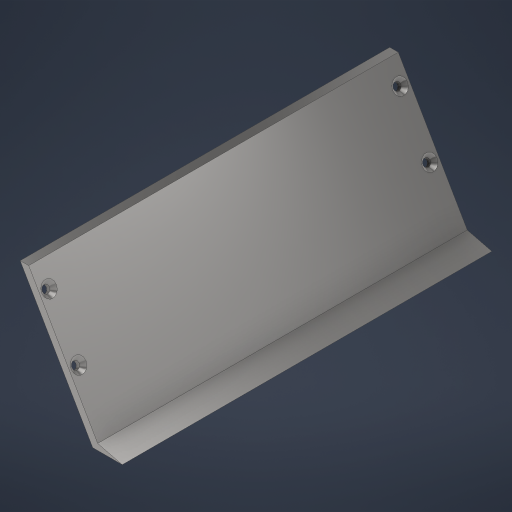
# Autodesk Inventor part: lemiesz
Saved by Autodesk Inventor 2024 (Build 280153000, 153)
## iProperties
Created: 2024-05-24
Part Number: lemiesz
Material: Steel
Document SubType Name: Modeling
Designer: Adam
Density: 7.85 g/cm^3
Appearance: Plate
Mass: 65.3515 g
Surface Area: 95.4294 cm^2
Volume: 8.32503 cm^3
Author: Adam
Autodesk Inventor part; units mm, degrees
ref_plane "YZ Plane" through (0, 0, 0) normal (1, 0, 0) x (0, 1, 0)
ref_plane "XZ Plane" through (0, 0, 0) normal (0, 1, 0) x (-1, 0, 0)
ref_plane "XY Plane" through (0, 0, 0) normal (0, 0, 1) x (1, 0, 0)
sketch "Sketch1" plane through (0, 0, 0) normal (0, 0, 1) x (1, 0, 0)
  line L0 (0, 0) -> (-8, 0)
  line L1 (-8, 0) -> (-27.6299, 34)
  line L2 (0, 0) -> (-6.6505, 1.6626)
  line L3 (-25.3205, 34) -> (-6.6505, 1.6626)
  line L4 (-27.6299, 34) -> (-25.3205, 34)
  dimension "d0" = 8
  dimension "d1" = 120
  dimension "d3" = 2
  constraints: 10 end point, 2 horizontal, 1 coincident, 1 parallel
  measures "d0" distance of L0.start L1.start
  measures "d1" angle of L0 L1
  measures "d3" distance between parallel lines of L3 L1
extrude "Extrusion1" add sketch "Sketch1" along normal mid plane 100
sketch "Sketch2" plane through (-25.3205, 34, 50) normal (0.8660254, 0.5, 0) x (0, 0, -1)
  line L0 (100, 0) -> (0, 0) projected
  point P0 (50, -42.1051)
  point P1 (2.5, -6)
  point P2 (2.5, -22)
  point P3 (97.5, -6)
  point P4 (97.5, -22)
hole "Hole1" at (-22.3205, 28.8038, 47.5) at (-14.3205, 14.9474, 47.5) at (-22.3205, 28.8038, -47.5) at (-14.3205, 14.9474, -47.5) direction (-0.8660254, -0.5, 0) diameter 2 end through all
chamfer "Chamfer1" distance 1 angle 45 4 edges at (-22.3205, 28.8038, 46.5) (-14.3205, 14.9474, 46.5) (-14.3205, 14.9474, -48.5) (-22.3205, 28.8038, -48.5) measured on face at (-22.3205, 28.8038, 46) measured on face at (-22.3205, 28.8038, -49) measured on face at (-14.3205, 14.9474, -49) measured on face at (-14.3205, 14.9474, 46)
body "Solid1"
